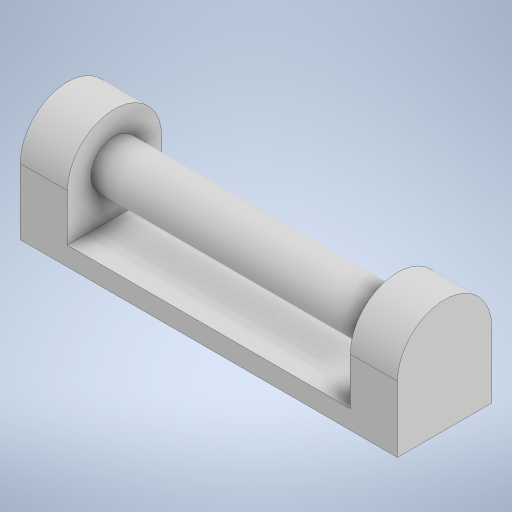
# Autodesk Inventor part: arm_base
Saved by Autodesk Inventor 2024.1 (Build 281209000, 209)
## iProperties
Created: 2025-01-27
Part Number: arm_base
Material: 一般
Document SubType Name: Modeling
Designer: hibik
Density: 1 g/cm^3
Appearance: 既定
Author: hibik
Autodesk Inventor part; units mm, degrees
ref_plane "YZ Plane" through (0, 0, 0) normal (1, 0, 0) x (0, 1, 0)
ref_plane "XZ Plane" through (0, 0, 0) normal (0, 1, 0) x (-1, 0, 0)
ref_plane "XY Plane" through (0, 0, 0) normal (0, 0, 1) x (1, 0, 0)
sketch "スケッチ1" plane through (0, 0, 0) normal (0, 1, 0) x (-1, 0, 0)
  line L0 (-15, -5) -> (15, -5)
  line L1 (15, -5) -> (15, 5)
  line L2 (15, 5) -> (-15, 5)
  line L3 (-15, 5) -> (-15, -5)
  line L4 (-15, -5) -> (15, 5) construction
  line L5 (15, -5) -> (-15, 5) construction
  point P0 (0, 0)
  dimension "d0" = 30
  dimension "d1" = 10
  constraints: 12 end point, 2 midpoint, 2 parallel, 1 horizontal, 1 perpendicular
  measures "d0" distance of L0.start L0.end
  measures "d1" distance of L0.end L1.end
extrude "押し出し1" add sketch "スケッチ1" along normal blind 2
sketch "スケッチ2" plane through (15, 0, 5) normal (1, 0, 0) x (0, 0, -1)
  circle A0 centre (5, 7) radius 2.5
  circle A1 centre (5, 7) radius 5
  line L0 (0, 2) -> (10, 2) projected
  line L1 (10, 0) -> (10, 2) projected
  line L2 (0, 0) -> (0, 2) projected
  line L3 (0, 2) -> (0, 7)
  line L4 (10, 2) -> (10, 7)
  line L5 (0, 0) -> (10, 0) projected
  point P0 (5, 0)
  dimension "d4" = 5
  constraints: 5 tangent, 4 end point, 2 centre point, 2 point on circle, 1 coincident
  measures "d4" diameter of A0
extrude "押し出し2" add sketch "スケッチ2" along normal blind 5
mirror "ミラー1" about plane through (0, 0, 0) normal (1, 0, 0) of "押し出し2"
sketch "スケッチ3" plane through (20, 0, 5) normal (1, 0, 0) x (0, 0, -1)
  circle A0 centre (5, 7) radius 2.5 projected
  point P0 (5, 0)
extrude "押し出し3" add sketch "スケッチ3" against normal up to surface (40 mm away)
